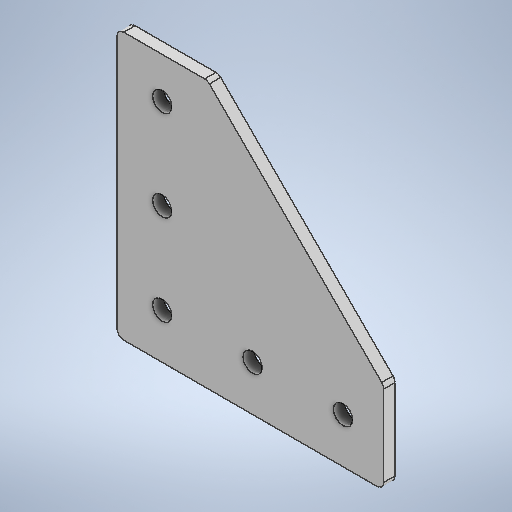
# Autodesk Inventor part: Connection_plate_L_120x120
Saved by Autodesk Inventor 2025.3 (Build 293356000, 356)
## iProperties
Created: 2026-05-31
Part Number: Connection_plate_L_120x120
Material: Generic
Document SubType Name: Modeling
Designer: louis
Density: 1 g/cm^3
Appearance: Default
Author: louis
Autodesk Inventor part; units mm, degrees
ref_plane "YZ Plane" through (0, 0, 0) normal (1, 0, 0) x (0, 1, 0)
ref_plane "XZ Plane" through (0, 0, 0) normal (0, 1, 0) x (-1, 0, 0)
ref_plane "XY Plane" through (0, 0, 0) normal (0, 0, 1) x (1, 0, 0)
sketch "Sketch1" plane through (0, 0, 0) normal (0, 0, 1) x (1, 0, 0)
  circle A0 centre (0, 0) radius 4.25
  circle A1 centre (40, 0) radius 4.25
  circle A2 centre (80, 0) radius 4.25
  circle A3 centre (0, 40) radius 4.25
  circle A4 centre (0, 80) radius 4.25
  line L0 (0, 0) -> (0, 80) construction
  line L1 (0, 0) -> (80, 0) construction
  line L2 (-20, 98) -> (-20, -20)
  line L3 (-20, -20) -> (98, -20)
  line L4 (98, -20) -> (98, 98)
  line L5 (98, 98) -> (-20, 98)
  line L6 (20, 98) -> (98, 20)
  dimension "d0" = 8.5
  dimension "d1" = 8.5
  dimension "d2" = 8.5
  dimension "d3" = 8.5
  dimension "d4" = 8.5
  dimension "d5" = 80
  dimension "d6" = 80
  dimension "d7" = 118
  dimension "d8" = 118
  dimension "d9" = 20
  dimension "d10" = 20
  dimension "d11" = 40
  dimension "d12" = 40
  constraints: 14 end point, 5 centre point, 2 coincident, 2 midpoint, 2 parallel, 2 point on line, 2 vertical, 1 horizontal, 1 perpendicular
  measures "d0" diameter of A0
  measures "d1" diameter of A4
  measures "d2" diameter of A3
  measures "d3" diameter of A1
  measures "d4" diameter of A2
  measures "d5" distance of L0.start L1.end
  measures "d6" distance of L0.start L0.end
  measures "d7" distance of L2.start L2.end
  measures "d8" distance of L2.end L3.end
  measures "d9" distance between parallel lines of L2 L0
  measures "d10" distance between parallel lines of L3 L1
  measures "d11" distance of L2.start L6.start
  measures "d12" distance of L3.end L6.end
extrude "Extrusion1" add sketch "Sketch1" along normal mid plane 5 contours L5 L6 L4 L3 L2
fillet "Fillet1" radius 3 5 edges at (-20, 98, 0) (20, 98, 0) (-20, -20, 0) (98, 20, 0) (98, -20, 0)
equation "\"d1\" = d0"
equation "\"d2\" = d0"
equation "\"d3\" = d0"
equation "\"d4\" = d0"
equation "\"d6\" = d5"
body "Solid1"
